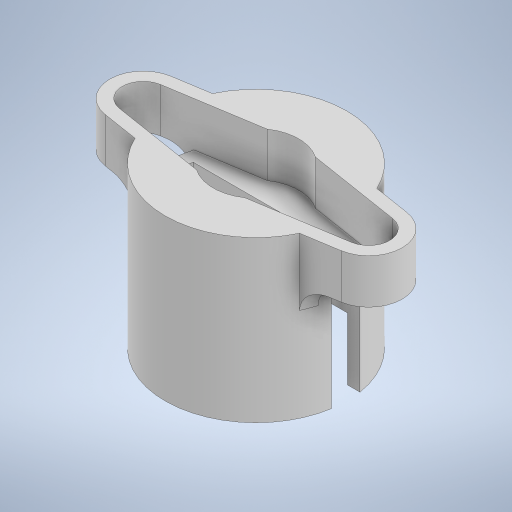
# Autodesk Inventor part: Handle Servo Interface
Saved by Autodesk Inventor 2023 (Build 270158000, 158)
## iProperties
Created: 2023-03-14
Part Number: Handle Servo Interface
Material: Generic
Document SubType Name: Modeling
Designer: tommy
Density: 1 g/cm^3
Appearance: Default
Author: tommy
Autodesk Inventor part; units mm, degrees
ref_plane "YZ Plane" through (0, 0, 0) normal (1, 0, 0) x (0, 1, 0)
ref_plane "XZ Plane" through (0, 0, 0) normal (0, 1, 0) x (-1, 0, 0)
ref_plane "XY Plane" through (0, 0, 0) normal (0, 0, 1) x (1, 0, 0)
sketch "Sketch1" plane through (0, 0, 0) normal (0, 1, 0) x (-1, 0, 0)
  circle A0 centre (0, 0) radius 11.176
  circle A1 centre (0, 0) radius 12.954
  line L0 (12.954, 0) -> (-12.954, 0)
  line L1 (12.954, -2.032) -> (-12.954, -2.032)
  line L2 (12.954, 2.032) -> (-12.954, 2.032)
  line L3 (3.4428, -5.0307) -> (16.5417, -2.9403)
  line L4 (3.4428, 5.0307) -> (16.5417, 2.9403)
  arc A2 (16.5417, -2.9403) -> (16.5417, 2.9403) centre (16.0725, 0) ccw
  line L5 (0, 12.954) -> (0, -12.954)
  line L6 (-3.4428, -5.0307) -> (-16.5417, -2.9403)
  line L7 (-3.4428, 5.0307) -> (-16.5417, 2.9403)
  arc A3 (-16.5417, 2.9403) -> (-16.5417, -2.9403) centre (-16.0725, 0) ccw
  line L8 (16.823, -4.7025) -> (3.7437, -6.7898)
  arc A4 (0, -7.7535) -> (3.7437, -6.7898) centre (0, 0) ccw
  arc A5 (-3.7437, -6.7898) -> (0, -7.7535) centre (0, 0) ccw
  line L9 (-3.7437, -6.7898) -> (-16.823, -4.7025)
  arc A6 (-16.823, 4.7025) -> (-16.823, -4.7025) centre (-16.0725, 0) ccw
  line L10 (-16.823, 4.7025) -> (-3.7437, 6.7898)
  arc A7 (0, 7.7535) -> (-3.7437, 6.7898) centre (0, 0) ccw
  arc A8 (3.7437, 6.7898) -> (0, 7.7535) centre (0, 0) ccw
  line L11 (3.7437, 6.7898) -> (16.823, 4.7025)
  arc A9 (16.823, -4.7025) -> (16.823, 4.7025) centre (16.0725, 0) ccw
  circle A10 centre (0, 0) radius 20.8345
  circle A11 centre (0, 0) radius 6.096
  point P0 (-10.9897, -2.032)
  point P1 (-12.7936, -2.032)
  point P2 (-12.7936, 2.032)
  point P3 (-10.9897, 2.032)
  point P4 (10.9897, 2.032)
  point P5 (10.9897, -2.032)
  point P6 (-20.8345, 0)
  point P7 (20.8345, 0)
  point P8 (-12.4454, -3.594)
  point P9 (-12.4454, 3.594)
  point P10 (12.4454, 3.594)
  point P11 (12.4454, -3.594)
  point P12 (11.7206, 5.5168)
  point P13 (-11.7206, 5.5168)
  point P14 (-11.7206, -5.5168)
  point P15 (11.7206, -5.5168)
  point P16 (10.47, -3.9093)
  point P17 (10.47, 3.9093)
  point P18 (-10.47, 3.9093)
  point P19 (-10.47, -3.9093)
  dimension "d0" = 22.352
  dimension "d1" = 25.908
  dimension "d3" = 2.032
  dimension "d8" = 2.032
  dimension "d18" = 12.192
  constraints: 24 end point, 24 point on circle, 12 centre point, 4 coincident, 3 symmetric about line, 2 parallel, 2 tangent, 1 horizontal, 1 vertical, 1 other
  measures "d0" diameter of A0
  measures "d1" diameter of A1
  measures "d3" distance between parallel lines of L0 L2
  measures "d8" distance between parallel lines of L1 L0
  measures "d18" diameter of A11
extrude "Extrusion1" add sketch "Sketch1" against normal blind 8.89 contours L0 A1 L1 A0 | A0 L2 A1 L0 | A0 L4 A1 L2 | L1 A1 L3 A0 | A0 L11 A1 L4 | L3 A1 L8 A0 | A0 L5 A1 L11 | L8 A1 L5 A0 | A0 L10 A1 L5 | L5 A1 L9 A0 | A0 L7 A1 L10 | L2 A1 L7 A0 | L9 A1 L6 A0 | A0 L6 A1 L1 picked at (11.6255, -1.8076) picked at (11.6255, 1.8076)
extrude "Extrusion2" add sketch "Sketch1" along normal blind 7.62 contours L0 A1 L1 A0 | A0 L2 A1 L0 | L2 A11 L4 A0 | A0 L4 A1 L2 | L1 A1 L3 A0 | A0 L3 A11 L1 | L4 A11 L5 A8 L11 A0 | A0 L11 A1 L4 | L2 L5 A11 | L3 A1 L8 A0 | A0 L8 A4 L5 A11 L3 | A11 L5 L1 | L11 A8 L5 A0 | A0 L5 A1 L11 | L2 A11 L5 | L8 A1 L5 A0 | A0 L5 A4 L8 | L5 A11 L1 | L5 A7 L10 A0 | A0 L10 A1 L5 | A11 L7 A0 L10 A7 L5 | L2 A0 L7 A11 | L5 A1 L9 A0 | A0 L9 A5 L5 | L5 A5 L9 A0 L6 A11 | A11 L6 A0 L1 | A0 L7 A1 L10 | L2 A1 L7 A0 | L9 A1 L6 A0 | A0 L6 A1 L1 picked at (11.6255, -1.8076) picked at (11.6255, 1.8076)
extrude "Extrusion3" add sketch "Sketch1" along normal blind 13.97 contours L4 A11 L5 A8 L11 A0 | A0 L11 A1 L4 | L3 A1 L8 A0 | A0 L8 A4 L5 A11 L3 | L11 A8 L5 A0 | A0 L5 A1 L11 | A1 L11 A9 L8 L3 A2 L4 | L8 A1 L5 A0 | A0 L5 A4 L8 | L5 A7 L10 A0 | A0 L10 A1 L5 | A11 L7 A0 L10 A7 L5 | L5 A1 L9 A0 | A0 L9 A5 L5 | L5 A5 L9 A0 L6 A11 | A0 L7 A1 L10 | L9 A1 L6 A0 | A1 L7 A3 L6 L9 A6 L10
extrude "Extrusion4" cut sketch "Sketch1" along normal up to surface (7.62 mm away) contours A1 L11 A9 L8 L3 A2 L4 | A1 L10 A6 A10 A9 L11 | L8 A9 A10 A6 L9 A1 | A1 L7 A3 L6 L9 A6 L10
fillet "Fillet1" radius 3.175 4 edges at (12.1212, 7.62, -4.5698) (12.1212, 7.62, 4.5698) (-12.1212, 7.62, 4.5698) (-12.1212, 7.62, -4.5698)
body "Solid1"
